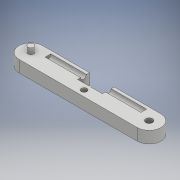
# Autodesk Inventor part: 1fjärdedel
Saved by Autodesk Inventor 2018 (Build 220112000, 112)
## iProperties
Created: 2018-02-08
Part Number: 1fjärdedel
Material: Generic
Document SubType Name: Modeling
Designer: davton
Density: 1 g/cm^3
Appearance: Default
Author: davton
Autodesk Inventor part; units mm, degrees
ref_plane "YZ Plane" through (0, 0, 0) normal (1, 0, 0) x (0, 1, 0)
ref_plane "XZ Plane" through (0, 0, 0) normal (0, 1, 0) x (-1, 0, 0)
ref_plane "XY Plane" through (0, 0, 0) normal (0, 0, 1) x (1, 0, 0)
sketch "Sketch1" plane through (0, 0, 0) normal (0, 0, 1) x (1, 0, 0)
  line L0 (-41.6667, 0) -> (41.6667, 0) construction
  line L1 (-41.6667, -8.3333) -> (41.6667, -8.3333)
  arc A0 (-41.6667, 8.3333) -> (-41.6667, -8.3333) centre (-41.6667, 0) ccw
  arc A1 (41.6667, -8.3333) -> (41.6667, 8.3333) centre (41.6667, 0) ccw
  line L2 (-8.75, 8.3333) -> (-41.6667, 8.3333)
  circle A2 centre (0, -4.1667) radius 2
  line L3 (0, 0) -> (-8.75, 0)
  line L4 (-8.75, 0) -> (-8.75, 8.3333)
  line L5 (0, 0) -> (8.75, 0)
  line L6 (8.75, 0) -> (8.75, 8.3333)
  line L7 (8.75, 8.3333) -> (41.6667, 8.3333)
  dimension "HL" = 41.6667
  dimension "d1" = 16.6667
  dimension "d10" = 4.1667
  dimension "HD" = 4
  dimension "d12" = 41.6667
  dimension "d13" = 8.75
  dimension "d14" = 8.75
  dimension "d17" = 8.75
  dimension "d18" = 8.3333
  constraints: 18 end point, 4 point on circle, 4 tangent, 3 centre point, 2 perpendicular, 2 point on line, 1 horizontal, 1 midpoint, 1 parallel
  measures "HL" distance of L3.start L0.end
  measures "d1" diameter of A1
  measures "d10" distance of L3.start A2.centre
  measures "HD" diameter of A2
  measures "d12" horizontal distance of L1.end A2.centre
  measures "d13" horizontal distance of L3.start L2.start
  measures "d14" distance of L3.start L3.end
  measures "d17" distance of L3.start L5.end
  measures "d18" distance of L5.end L6.end
extrude "Main" add sketch "Sketch1" along normal blind 8.3333
sketch "Sketch2" plane through (-8.75, 0, 0) normal (1, 0, 0) x (0, 0, -1)
  line L0 (-8.3333, 8.3333) -> (-8.3333, 0) projected
  circle A0 centre (-8.3333, 4.1667) radius 2
  point P0 (0, 0)
  dimension "d19" = 4
  constraints: 1 centre point, 1 midpoint
  measures "d19" diameter of A0
extrude "Hole" cut sketch "Sketch2" along normal blind 42.5 and the other way blind 25
sketch "Sketch3" plane through (0, 0, 8.3333) normal (0, 0, 1) x (1, 0, 0)
  circle A0 centre (-41.6667, 0) radius 2
  line L0 (41.6667, 8.3333) -> (8.75, 8.3333) projected
  line L1 (-8.75, 8.3333) -> (-41.6667, 8.3333) projected
  point P0 (0, 0)
  dimension "d24" = 4
  dimension "d25" = 41.6667
  dimension "d29" = 8.3333
  constraints: 1 centre point
  measures "d24" diameter of A0
  measures "d25" distance of point (0, 0) A0.centre
  measures "d29" distance from line of L1 A0.centre
sketch "Sketch4" plane through (0, 0, 8.3333) normal (0, 0, 1) x (1, 0, 0)
  circle A0 centre (41.6667, 0) radius 2.4167
  line L0 (41.6667, 8.3333) -> (8.75, 8.3333) projected
  point P0 (0, 0)
  dimension "d30" = 41.6667
  dimension "d31" = 4.8333
  dimension "d32" = 8.3333
  constraints: 1 centre point
  measures "d30" distance of A0.centre point (0, 0)
  measures "d31" diameter of A0
  measures "d32" distance from line of L0 A0.centre
extrude "Pigg" add sketch "Sketch3" along normal blind 4.1667
extrude "Minuspigg" cut sketch "Sketch4" against normal blind 4.1667
sketch "Sketch5" plane through (0, 0, 8.3333) normal (0, 0, 1) x (1, 0, 0)
  point P0 (0, 0)
sketch "Sketch6" plane through (0, 0, 8.3333) normal (0, 0, 1) x (1, 0, 0)
  point P0 (0, 0)
sketch "Sketch7" plane through (0, 0, 8.3333) normal (0, 0, 1) x (1, 0, 0)
  point P0 (0, 0)
sketch "Sketch8" plane through (0, 0, 8.3333) normal (0, 0, 1) x (1, 0, 0)
  point P0 (0, 0)
sketch "Sketch9" plane through (0, 0, 8.3333) normal (0, 0, 1) x (1, 0, 0)
  point P0 (0, 0)
equation "\"d1\" = 0.4 * HL"
equation "\"d10\" = 0.1 * HL"
equation "\"d12\" = HL"
equation "\"d13\" = 0.2 * HL + Eps"
equation "\"d14\" = 0.2 * HL + Eps"
equation "\"d17\" = 0.2 * HL + Eps"
equation "\"d18\" = 0.2 * HL"
equation "\"d15\" = 0.2 * HL"
equation "\"d19\" = HD"
equation "\"d20\" = HL + 2 * Eps"
equation "\"d21\" = 0.6 * HL"
equation "\"d24\" = HD"
equation "\"d25\" = HL"
equation "\"d29\" = 0.2 * HL"
equation "\"d30\" = HL"
equation "\"d31\" = HD + 2 * Eps"
equation "\"d32\" = 0.2 * HL"
equation "\"d33\" = 0.1 * HL"
equation "\"d35\" = 0.1 * HL"
equation "\"Eps\" = 0.41667"
body "Solid1"
